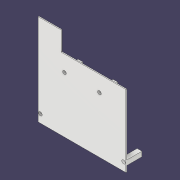
# Autodesk Inventor part: BP013
Saved by Autodesk Inventor 2017 SP1 (Build 210196100, 196)
## iProperties
Created: 2018-06-20
Part Number: BP013
Material: ABS Plastic
Document SubType Name: Modeling
Designer: Zach
Density: 1.06 g/cm^3
Appearance: CR White
Author: Zach
Autodesk Inventor part; units mm, degrees
ref_plane "YZ Plane" through (0, 0, 0) normal (1, 0, 0) x (0, 1, 0)
ref_plane "XZ Plane" through (0, 0, 0) normal (0, 1, 0) x (-1, 0, 0)
ref_plane "XY Plane" through (0, 0, 0) normal (0, 0, 1) x (1, 0, 0)
sketch "Sketch1" plane through (0, 0, 0) normal (0, 0, 1) x (1, 0, 0)
  circle A0 centre (0, 0) radius 2.5
  circle A1 centre (109.2883, 0) radius 2.5
  line L0 (-82.8559, 30) -> (192.1441, 30)
  line L1 (192.1441, 30) -> (192.1441, -175)
  line L2 (192.1441, -175) -> (-82.8559, -175)
  line L3 (-82.8559, -175) -> (-82.8559, 30)
  line L4 (0, 0) -> (109.2883, 0) construction
  point P0 (54.6441, 0)
  point P1 (54.6441, 30)
  dimension "d0" = 5
  dimension "d1" = 5
  dimension "d2" = 109.2883
  dimension "d3" = 275
  dimension "d4" = 30
  dimension "d5" = 175
  constraints: 10 end point, 2 centre point, 2 horizontal, 2 midpoint, 2 parallel, 1 coincident, 1 horizontal alignment, 1 perpendicular, 1 vertical alignment
  measures "d0" diameter of A0
  measures "d1" diameter of A1
  measures "d2" distance of L4.end point (0, 0)
  measures "d3" distance of L1.end L2.end
  measures "d4" distance from line of L0 L4.end
  measures "d5" distance from line of L2 L4.end
extrude "Extrusion1" add sketch "Sketch1" along normal blind 3
sketch "Sketch4" plane through (0, 0, 0) normal (0, 0, -1) x (-1, 0, 0)
  circle A0 centre (-109.2883, 0) radius 2.5 projected
  line L0 (-116.7883, -7.5) -> (-101.7883, -7.5)
  line L1 (-101.7883, -7.5) -> (-101.7883, 7.5)
  line L2 (-101.7883, 7.5) -> (-116.7883, 7.5)
  line L3 (-116.7883, 7.5) -> (-116.7883, -7.5)
  circle A1 centre (-109.2883, 0) radius 2.5 projected
  line L4 (-116.7883, -7.5) -> (-101.7883, 7.5) construction
  line L5 (-101.7883, -7.5) -> (-116.7883, 7.5) construction
  line L6 (7.5, -7.5) -> (-7.5, -7.5)
  line L7 (-7.5, -7.5) -> (-7.5, 7.5)
  line L8 (-7.5, 7.5) -> (7.5, 7.5)
  line L9 (7.5, 7.5) -> (7.5, -7.5)
  circle A2 centre (0, 0) radius 2.5 projected
  line L10 (7.5, -7.5) -> (-7.5, 7.5) construction
  line L11 (-7.5, -7.5) -> (7.5, 7.5) construction
  dimension "d14" = 15
  dimension "d15" = 15
  dimension "d16" = 15
  dimension "d17" = 15
  constraints: 24 end point, 4 midpoint, 4 parallel, 2 horizontal, 2 perpendicular
  measures "d14" distance of L2.end L1.end
  measures "d15" distance of L1.end L0.end
  measures "d16" distance of L7.end L8.end
  measures "d17" distance of L6.end L7.end
extrude "Extrusion4" add sketch "Sketch4" along normal blind 47
sketch "Sketch5" plane through (0, 0, 3) normal (0, 0, 1) x (1, 0, 0)
  circle A0 centre (0, 0) radius 2.5 projected
  circle A1 centre (109.2883, 0) radius 2.5 projected
  circle A2 centre (0, 0) radius 5.5
  circle A3 centre (109.2883, 0) radius 5.5
  dimension "d20" = 11
  dimension "d21" = 11
  constraints: 2 centre point, 2 coincident
  measures "d20" diameter of A2
  measures "d21" diameter of A3
extrude "Extrusion5" cut sketch "Sketch5" against normal blind 47
sketch "Sketch6" plane through (0, 0, 0) normal (0, 0, -1) x (-1, 0, 0)
  line L0 (-192.1441, 30) -> (-192.1441, -175) projected
  line L1 (-192.1441, -157) -> (-177.1441, -157)
  line L2 (-177.1441, -157) -> (-177.1441, -142)
  line L3 (-177.1441, -142) -> (-192.1441, -142)
  line L4 (-192.1441, -142) -> (-192.1441, -157)
  line L5 (82.8559, -175) -> (82.8559, 30) projected
  line L6 (82.8559, -157) -> (67.8559, -157)
  line L7 (67.8559, -157) -> (67.8559, -142)
  line L8 (67.8559, -142) -> (82.8559, -142)
  line L9 (82.8559, -142) -> (82.8559, -157)
  line L10 (-192.1441, -175) -> (82.8559, -175) projected
  point P0 (0, 0)
  dimension "d24" = 15
  dimension "d25" = 15
  dimension "d26" = 15
  dimension "d27" = 15
  dimension "d28" = 18
  constraints: 16 end point, 4 parallel, 3 point on line, 2 horizontal, 2 perpendicular
  measures "d24" distance of L3.end L2.end
  measures "d25" distance of L2.end L1.end
  measures "d26" distance of L7.end L8.end
  measures "d27" distance of L6.end L7.end
  measures "d28" distance between parallel lines of L10 L1
extrude "Extrusion6" add sketch "Sketch6" along normal blind 47
sketch "Sketch7" plane through (0, 0, 3) normal (0, 0, 1) x (1, 0, 0)
  line L0 (-10.3559, 30) -> (-82.8559, 30)
  line L1 (-82.8559, 30) -> (-10.3559, 30)
  line L2 (-10.3559, 30) -> (-10.3559, 110)
  line L3 (-10.3559, 110) -> (-82.8559, 110)
  line L4 (-82.8559, 110) -> (-82.8559, 30)
  line L5 (-82.8559, 30) -> (-82.8559, -175) projected
  point P0 (0, 0)
  dimension "d31" = 80
  dimension "d42" = 72.5
  constraints: 10 end point, 2 parallel, 1 horizontal, 1 perpendicular
  measures "d31" distance of L0.start L2.end
  measures "d42" distance of L2.end L3.end
extrude "Extrusion7" add sketch "Sketch7" against normal blind 3
sketch "Sketch8" plane through (0, 0, -47) normal (0, 0, -1) x (-1, 0, 0)
  line L0 (-192.1441, -157) -> (-177.1441, -157) projected
  line L1 (-177.1441, -157) -> (-177.1441, -142) projected
  line L2 (-177.1441, -142) -> (-192.1441, -142) projected
  line L3 (-192.1441, -142) -> (-192.1441, -157) projected
  line L4 (82.8559, -157) -> (82.8559, -142) projected
  line L5 (82.8559, -142) -> (67.8559, -142) projected
  line L6 (67.8559, -142) -> (67.8559, -157) projected
  line L7 (67.8559, -157) -> (82.8559, -157) projected
  circle A0 centre (-184.6441, -149.5) radius 2.5
  circle A1 centre (75.3559, -149.5) radius 2.5
  point P0 (0, 0)
  point P1 (75.3559, -157)
  point P2 (-184.6441, -157)
  point P3 (-177.1441, -149.5)
  point P4 (67.8559, -149.5)
  dimension "d34" = 5
  dimension "d35" = 5
  constraints: 4 midpoint, 2 centre point, 2 horizontal alignment, 2 vertical alignment
  measures "d34" diameter of A0
  measures "d35" diameter of A1
extrude "Extrusion8" cut sketch "Sketch8" against normal through all contours A0 | A1
sketch "Sketch9" plane through (0, 0, 3) normal (0, 0, 1) x (1, 0, 0)
  circle A0 centre (-75.3559, -149.5) radius 2.5 projected
  circle A1 centre (184.6441, -149.5) radius 2.5 projected
  circle A2 centre (-75.3559, -149.5) radius 5.5
  circle A3 centre (184.6441, -149.5) radius 5.5
  point P0 (0, 0)
  dimension "d38" = 11
  dimension "d39" = 11
  constraints: 2 centre point, 2 coincident
  measures "d38" diameter of A2
  measures "d39" diameter of A3
extrude "Extrusion9" cut sketch "Sketch9" against normal blind 47
sketch "Sketch10" plane through (0, 0, 3) normal (0, 0, 1) x (1, 0, 0)
  line L0 (192.1441, 30) -> (-10.3559, 30) projected
  line L1 (-10.3559, 30) -> (-10.3559, 110) projected
  line L2 (-10.3559, 30) -> (192.1441, 30) projected
  line L3 (-10.3559, 110) -> (-10.3559, 30) projected
  line L4 (192.1441, 30) -> (-10.3559, 30)
  line L5 (-10.3559, 30) -> (-10.3559, 50)
  line L6 (-10.3559, 50) -> (192.1441, 50)
  line L7 (192.1441, 50) -> (192.1441, 30)
  point P0 (0, 0)
  dimension "d43" = 20
  constraints: 8 end point, 2 parallel, 1 horizontal, 1 perpendicular, 1 point on line
  measures "d43" distance of L6.end L0.start
extrude "Extrusion10" add sketch "Sketch10" against normal blind 3
body "Solid1"
